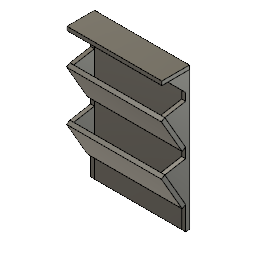
MailOrganizer (Autodesk Fusion 360 design; units mm, degrees)
Autodesk Fusion 360 part; units mm, degrees
sketch "Sketch1" plane through (0, 0, 0) normal (1, 0, 0) x (0, 0, -1)
  line L0 (0, 0) -> (0, 444.5)
  line L1 (0, 444.5) -> (-12.7, 444.5)
  line L2 (-12.7, 444.5) -> (-12.7, 0)
  line L3 (-12.7, 0) -> (0, 0)
  line L4 (0, 444.5) -> (-88.9, 444.5)
  line L5 (-88.9, 444.5) -> (-88.9, 457.2)
  line L6 (-88.9, 457.2) -> (0, 457.2)
  line L7 (0, 457.2) -> (0, 444.5)
  line L8 (-69.85, 444.5) -> (-12.7, 387.35)
  line L9 (-12.7, 76.2) -> (-79.375, 191.6845)
  line L10 (-79.375, 191.6845) -> (-12.7, 203.4411)
  line L11 (-12.7, 235.4) -> (-79.375, 350.8845)
  line L12 (-79.375, 350.8845) -> (-12.7, 362.6411)
  line L13 (-79.375, 191.6845) -> (-90.3735, 185.3345)
  line L14 (-90.3735, 185.3345) -> (-12.7, 50.8)
  line L15 (-79.375, 350.8845) -> (-90.3735, 344.5345)
  line L16 (-90.3735, 344.5345) -> (-12.7, 210)
  line L17 (-12.7, 76.2) -> (-23.6985, 69.85)
  line L18 (-12.7, 235.4) -> (-23.6985, 229.05)
  line L19 (0, 0) -> (0.4, 0)
  line L20 (0.4, 0) -> (0.4, 457.2)
  line L21 (0.4, 457.2) -> (0, 457.2)
  dimension "d5" = 12.7
  dimension "d6" = 457.2
  dimension "d7" = 12.7
  dimension "d8" = 88.9
  dimension "d9" = 45
  dimension "d10" = 19.05
  dimension "d11" = 30
  dimension "d12" = 80
  dimension "d13" = 12.7
  dimension "d15" = 133.35
  dimension "d16" = 50.8
  dimension "d17" = 210
  dimension "d100" = 0.4
  measures "d6" distance of L3 L6
  measures "d7" distance of L0.start
  measures "d9" angle of L0 L8
  measures "d11" angle of L0 L9
  measures "d12" angle of L0 L10
  measures "d15" distance of L0.start
  measures "d16" distance of L3
  measures "d17" distance of L3
  measures "d100" distance of L0 L20
extrude "Extrude1" add sketch "Sketch1" along normal blind 12.7 contours L0 L1 L2 L3 L4 | L0 L7 L19 L20 L21 | L2 L4 L8 | L2 L9 L10 | L2 L11 L12 makes body 1 in component "Left End"
extrude "Extrude1'" add sketch "Sketch1" along normal blind 279.4 from surface at 12.7 separate body contours L0 L1 L2 L3 L4 makes body 2 in component "Back"
extrude "Extrude1''" add sketch "Sketch1" along normal blind 12.7 from surface at 292.1 separate body contours L0 L1 L2 L3 L4 | L0 L7 L19 L20 L21 | L2 L4 L8 | L2 L9 L10 | L2 L11 L12 makes body 3 in component "Right End"
extrude "Extrude1'''" add sketch "Sketch1" along normal blind 304.8 separate body contours L1 L4 L5 L6 L7 makes body 4 in component "Shelf"
extrude "Extrude1''''" add sketch "Sketch1" along normal blind 304.8 separate body contours L11 L15 L16 L18 makes body 5 in component "Top Cubbie"
extrude "Extrude1'''''" add sketch "Sketch1" along normal blind 304.8 separate body contours L9 L13 L14 L17 makes body 6 in component "Bottom Cubbie"
component "Left End" placed x (1, 0, 0) y (0, 1, 0) z (0, 0, 1) at (0, 0, 0)
component "Back" placed x (1, 0, 0) y (0, 1, 0) z (0, 0, 1) at (0, 0, 0)
component "Right End" placed x (1, 0, 0) y (0, 1, 0) z (0, 0, 1) at (0, 0, 0)
component "Shelf" placed x (1, 0, 0) y (0, 1, 0) z (0, 0, 1) at (0, 0, 0)
component "Top Cubbie" placed x (1, 0, 0) y (0, 1, 0) z (0, 0, 1) at (0, 0, 0)
component "Bottom Cubbie" placed x (1, 0, 0) y (0, 1, 0) z (0, 0, 1) at (0, 0, 0)
equation "Ply1 = 18 mm" comment "3/4\" Plywood thickness"
equation "Height = 18 in"
equation "Width = 12 in"
equation "Ply2 = 12.7 mm" comment "1/2\" Plywood thickness"
equation "d5 = Ply2"
equation "d6 = Height"
equation "d7 = Ply2"
equation "d13 = Ply2"
equation "d18 = Ply2"
equation "Dado = 6.35 mm" comment "Dado Depth"
equation "Clr = 0.4 mm" comment "Clearance Distance"
equation "d29 = Width - ( 2 * Ply2 )"
equation "d32 = Ply2"
equation "d34 = Width"
equation "d36 = Width"
equation "d38 = Width"
equation "d100 = Clr"
